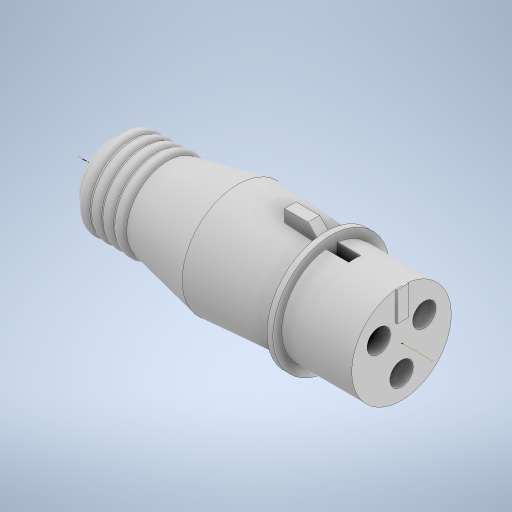
# Autodesk Inventor part: finalproject2
Saved by Autodesk Inventor 2023 (Build 270158000, 158)
## iProperties
Created: 2023-10-24
Part Number: finalproject2
Material: Generic
Document SubType Name: Modeling
Designer: Rahul
Density: 1 g/cm^3
Appearance: Default
Author: Rahul
Autodesk Inventor part; units mm, degrees
sketch "Sketch1" plane through (0, 0, 0) normal (0, 1, 0) x (-1, 0, 0)
  line L0 (0, 0) -> (0, -8.5)
  line L1 (0, -8.5) -> (12, -8.5)
  line L2 (12, -8.5) -> (12, -10)
  line L3 (12, -10) -> (13, -10)
  line L4 (13, -10) -> (13, -8.5)
  line L5 (13, -8.5) -> (28, -9.5)
  line L6 (28, -9.5) -> (40, -7)
  line L7 (40, -7) -> (48, -7)
  line L8 (48, -7) -> (48, -6)
  line L9 (48, -6) -> (48.5, -6)
  line L10 (50, -4.5) -> (50, 0)
  line L11 (50, 0) -> (0, 0)
  arc A0 (48.5, -6) -> (50, -4.5) centre (48.5, -4.5) ccw
  point P0 (50, -6)
  dimension "d0" = 50
  dimension "d1" = 8.5
  dimension "d2" = 12
  dimension "d3" = 1.5
  dimension "d4" = 1
  dimension "d5" = 48
  dimension "d6" = 8
  dimension "d7" = 12
  dimension "d8" = 9.5
  dimension "d9" = 7
  dimension "d10" = 6
  dimension "d11" = 1.5
  constraints: 24 end point, 8 perpendicular, 3 point on line, 2 point on circle, 2 tangent, 1 centre point, 1 horizontal, 1 vertical
  measures "d0" distance between parallel lines of L0 L10
  measures "d1" distance of L0.start L0.end
  measures "d2" distance of L0.end L1.end
  measures "d3" distance of L1.end L2.end
  measures "d4" distance of L2.end L3.end
  measures "d5" distance between parallel lines of L0 L8
  measures "d6" distance of L6.end L7.end
  measures "d7" horizontal distance of L6.end L5.end
  measures "d8" distance from line of L5.end L11
  measures "d9" distance between parallel lines of L7 L11
  measures "d10" distance of point (50, -6) L10.end
  measures "d11" radius of A0
revolve "Revolution1" add sketch "Sketch1" angle 360 about axis through (-50, 0, 0) along (1, 0, 0)
ref_plane "Work Plane1" through (0, 0, 0) normal (1, 0, 0) x (0, 0, -1)
sketch "Sketch2" plane through (0, 0, 0) normal (1, 0, 0) x (0, 0, -1)
  circle A0 centre (0, 0) radius 8.5 projected
  line L0 (1.0056, 8.4416) -> (1.0056, 3.4416)
  line L1 (-0.9944, 8.4416) -> (-0.9944, 3.4416)
  line L2 (-0.9944, 3.4416) -> (1.0056, 3.4416)
  arc A1 (1.0056, 8.4416) -> (-0.9944, 8.4301) centre (0.0504, 0.6774) ccw
  point P0 (1.0056, 8.4403)
  point P1 (0, 8.5)
  dimension "d14" = 5
  dimension "d16" = 5
  dimension "d17" = 2
  constraints: 6 end point, 2 point on circle, 2 vertical, 1 centre point, 1 horizontal, 1 point on line, 2 other
  measures "d14" distance of L0.start L0.end
  measures "d16" distance of L1.start L1.end
  measures "d17" distance between parallel lines of L1 L0
extrude "Extrusion1" add sketch "Sketch2" along normal blind 0.25 contours L0 L2 L1 A1 A0
ref_plane "Work Plane2" through (0, 3.4416, -1.0056) normal (1, 0, 0) x (0, 0, -1)
sketch "Sketch3" plane through (0, 3.4416, -1.0056) normal (1, 0, 0) x (0, 0, -1)
  circle A0 centre (-1.0056, -3.4416) radius 4.5 projected
  point P0 (-1.0056, -7.9416)
  point P1 (-1.0056, -7.9416)
  point P2 (-1.0056, -7.9416)
  point P3 (2.8906, -1.1663)
  point P4 (-4.9018, -1.1663)
  constraints: 2 coincident, 1 vertical alignment, 1 other
hole "Hole1" at (0, -4.5, 0) at (0, -4.5, 0) at (0, 2.2754, -3.8962) at (0, 2.2754, 3.8962) direction (-1, 0, 0) diameter 4 depth 4
ref_plane "Work Plane3" through (-19, 0, 0) normal (-1, 0, 0) x (0, 0, 1)
sketch "Sketch4" plane through (-19, 0, 0) normal (-1, 0, 0) x (0, 0, 1)
  circle A0 centre (0, 0) radius 8.9031
  line L0 (0, 8.9031) -> (1, 8.9031)
  line L1 (0, 8.9031) -> (-1, 8.9031)
  line L2 (1, 8.9031) -> (-1, 8.9031)
  line L3 (-1, 8.9031) -> (-1, 10.9031)
  line L4 (-1, 10.9031) -> (1, 10.9031)
  line L5 (1, 10.9031) -> (1, 8.9031)
  line L6 (1, 8.9031) -> (-1, 8.9031)
  dimension "d29" = 1
  dimension "d30" = 1
  dimension "d31" = 2
  constraints: 14 end point, 4 horizontal, 2 parallel, 1 coincident, 1 perpendicular, 1 vertical alignment, 2 other
  measures "d29" distance of L0.start L0.end
  measures "d30" distance of L0.start L1.end
  measures "d31" distance of L2.end L3.end
extrude "Extrusion2" add sketch "Sketch4" against normal blind 4 contours L1 L3 L4 L5 L0
sketch "Sketch5" plane through (-19, 8.9031, 1) normal (0, 0, 1) x (1, 0, 0)
  line L0 (4, 2) -> (4, 0) projected
  line L1 (4, 0) -> (6, 0)
  line L2 (6, 0) -> (4, 2)
  point P0 (19, -8.9031)
  dimension "d34" = 2
  constraints: 4 end point, 1 horizontal
  measures "d34" distance of L0.end L1.end
extrude "Extrusion3" add sketch "Sketch5" against normal up to surface (2 mm away)
sketch "Sketch6" plane through (-19, 8.9031, -1) normal (0, -1, 0) x (1, 0, 0)
  line L0 (0, 0) -> (6, 0) projected
  line L1 (6, 0) -> (0, 0)
  line L2 (0, 0) -> (0, 2)
  line L3 (0, 2) -> (6, 2)
  line L4 (6, 2) -> (6, 0)
  point P0 (19, 1)
  constraints: 8 end point, 2 parallel, 1 horizontal, 1 perpendicular
extrude "Extrusion4" add sketch "Sketch6" along normal blind 1
ref_plane "Work Plane4" through (0, 8.5, 0) normal (0, 1, 0) x (-1, 0, 0)
sketch "Sketch7" plane through (0, 8.5, 0) normal (0, 1, 0) x (-1, 0, 0)
  line L0 (13, 1) -> (15, 1) projected
  line L1 (19, -1) -> (15, -1) projected
  line L2 (19, -1) -> (3.9639, -1)
  line L3 (19, 1) -> (15, 1) projected
  line L4 (19, 1) -> (4, 1)
  line L5 (4, 2) -> (4, -2) projected
  line L6 (8, 1) -> (8, -1)
  line L7 (12, 8.5) -> (12, -8.5) projected
  line L8 (12, 1) -> (12, -1)
  point P0 (0, 0)
  dimension "d39" = 4
  constraints: 8 end point, 7 point on line, 1 collinear, 1 horizontal, 1 perpendicular
  measures "d39" distance of L8.start L6.start
extrude "Extrusion5" cut sketch "Sketch7" against normal blind 2 contours L2 L6 L4 L7
ref_plane "Work Plane6" through (-6, 6.5, 0) normal (0, 1, 0) x (-1, 0, 0)
ref_plane "Work Plane5" through (-6, 8.5, 0) normal (0, 1, 0) x (-1, 0, 0)
sketch "Sketch8" plane through (-6, 6.5, 0) normal (0, 1, 0) x (-1, 0, 0)
  circle A0 centre (5.75, 0) radius 0.25
  line L0 (6, 1) -> (6, -1) projected
  line L1 (2, 1) -> (6, 1) projected
  line L2 (2, -1) -> (2, 1) projected
  line L3 (6, -1) -> (2, -1) projected
  line L4 (6, 1) -> (6, -1) projected
  point P0 (-6, 0)
  dimension "d43" = 0.5
  constraints: 1 centre point, 1 tangent
  measures "d43" diameter of A0
extrude "Extrusion6" cut sketch "Sketch8" against normal blind 1 contours A0
sketch "Sketch9" plane through (0, 6.5, 0) normal (0, 1, 0) x (1, 0, 0)
  circle A0 centre (-8.25, 0) radius 0.25
  line L0 (-8, -1) -> (-8, 1) projected
  point P0 (0, 0)
  dimension "d46" = 0.5
  constraints: 1 centre point, 1 tangent
  measures "d46" diameter of A0
extrude "Extrusion7" cut sketch "Sketch9" against normal blind 1
sketch "Sketch10" plane through (-6, 6.5, 0) normal (0, 1, 0) x (-1, 0, 0)
  point P0 (-6, 0)
sketch "Sketch11" plane through (0, 0, 0) normal (0, 1, 0) x (-1, 0, 0)
  line L0 (40, 7) -> (40, -7) projected
  circle A0 centre (41.001, 6.293) radius 1.2255
  circle A1 centre (43.1416, 6.1762) radius 1.2255
  circle A2 centre (47.1448, 6.293) radius 1.1096
  line L1 (42.0019, 7) -> (42.2343, 7)
  line L2 (48, 7) -> (40, 7) projected
  line L3 (48, 7) -> (40, 7) projected
  line L4 (48, 7) -> (40, 7) projected
  line L5 (45.6731, 7) -> (48, 7)
  line L6 (48, 7) -> (40, 7) projected
  line L7 (48, 7) -> (40, 7) projected
  line L8 (48, 7) -> (40, 7) projected
  line L9 (44.0489, 7) -> (44.522, 7)
  line L10 (48, 7) -> (40, 7) projected
  line L11 (41.001, 6.293) -> (47.1448, 6.293)
  line L12 (48, 7) -> (40, 7) projected
  circle A3 centre (45.1365, 6.293) radius 1.1096
  line L13 (44.0489, 7) -> (44.2813, 7)
  line L14 (48, 7) -> (40, 7) projected
  line L15 (48, 7) -> (40, 7) projected
  line L16 (45.9917, 7) -> (46.2896, 7)
  line L17 (48, 7) -> (40, 7) projected
  line L18 (45.9917, 7) -> (46.2896, 7)
  line L19 (46.2896, 7) -> (46.2896, 7.77)
  line L20 (46.2896, 7.77) -> (45.9917, 7.77)
  line L21 (45.9917, 7.77) -> (45.9917, 7)
  line L22 (42.0019, 7) -> (42.2343, 7)
  line L23 (48, 7) -> (40, 7) projected
  point P0 (0, 0)
  point P1 (45.9917, 7)
  constraints: 22 end point, 8 point on circle, 5 horizontal, 4 centre point, 2 equal radius, 2 parallel, 2 point on line, 1 collinear, 1 perpendicular, 18 other
ref_plane "Work Plane8" through (-44, 0, 0) normal (0, 1, 0) x (-1, 0, 0)
ref_plane "Work Plane7" through (-44, 7, 0) normal (0, 1, 0) x (-1, 0, 0)
sketch "Sketch12" plane through (-44, 0, 0) normal (0, 1, 0) x (-1, 0, 0)
  line L0 (-44, 0) -> (-44.25, 0) projected
  line L1 (-44.25, 0) -> (10.6438, 0)
  constraints: 2 end point, 1 horizontal
revolve "Revolution2" add sketch "Sketch11" angle 360 about axis through (0.25, 0, 0) along (-1, 0, 0) picked at (46.8413, 6.8183) contours A0 L2 | A1 L2 | A3 A2 L2 | A2 L11 A3 | A3 L2 | A2 A3 L11 | L2 A2
body "Solid1"
